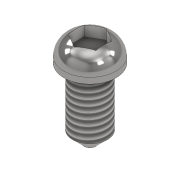
# Autodesk Inventor part: M3x6mm_screw
Saved by Autodesk Inventor 2020 (Build 240168000, 168)
## iProperties
Created: 2021-02-24
Part Number: M3x6mm_screw
Material: Generic
Document SubType Name: Modeling
Designer: JojoS
Density: 1 g/cm^3
Appearance: Default
Author: JojoS
Autodesk Inventor part; units mm, degrees
ref_plane "YZ Plane" through (0, 0, 0) normal (1, 0, 0) x (0, 1, 0)
sketch "Sketch1" plane through (0, 0, 0) normal (0, 1, 0) x (-1, 0, 0)
  circle A0 centre (0, 0) radius 1.5
  dimension "d0" = 3
  constraints: 1 centre point, 1 coincident
  measures "d0" diameter of A0
extrude "Extrusion1" add sketch "Sketch1" along normal blind 6
chamfer "Chamfer1" distance 1 angle 45 1 edges at (1.5, 0, 0)
ref_plane "Work Plane1" through (0, 6, 0) normal (0, 1, 0) x (1, 0, 0)
sketch "Sketch2" plane through (0, 6, 0) normal (0, 1, 0) x (1, 0, 0)
  circle A0 centre (0, 0) radius 0.5 projected
  circle A1 centre (0, 0) radius 2.25
  dimension "d7" = 4.5
  constraints: 1 centre point, 1 coincident
  measures "d7" diameter of A1
extrude "Extrusion2" add sketch "Sketch2" along normal blind 2 contours A0 | A1
fillet "Fillet1" radius 1.5 1 edges at (-2.25, 8, 0)
ref_plane "Work Plane2" through (0, 8, 0) normal (0, 1, 0) x (1, 0, 0)
sketch "Sketch3" plane through (0, 8, 0) normal (0, 1, 0) x (1, 0, 0)
  line L0 (-1.2, 0.6928) -> (0, 1.3856)
  line L1 (0, 1.3856) -> (1.2, 0.6928)
  line L2 (1.2, 0.6928) -> (1.2, -0.6928)
  line L3 (1.2, -0.6928) -> (0, -1.3856)
  line L4 (0, -1.3856) -> (-1.2, -0.6928)
  line L5 (-1.2, -0.6928) -> (-1.2, 0.6928)
  point P0 (0, 0)
  point P1 (0, 0)
  dimension "d12" = 1.2
  constraints: 12 end point, 1 coincident, 13 other
  measures "d12" distance from line of point (0, 0) L5
extrude "Extrusion3" cut sketch "Sketch3" against normal blind 1
thread "Thread1" size "M3x0.5" class "6g" standard "ANSI Metric M Profile" full length
body "Solid1"
